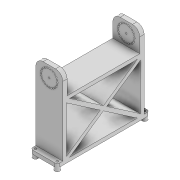
# Autodesk Inventor part: StereoVisionHolder
Saved by Autodesk Inventor 2022 (Build 260153000, 153)
## iProperties
Created: 2022-11-13
Part Number: StereoVisionHolder
Material: Generic
Document SubType Name: Modeling
Designer: MVeszpremi
Density: 1 g/cm^3
Appearance: Default
Author: MVeszpremi
Autodesk Inventor part; units mm, degrees
ref_plane "YZ Plane" through (0, 0, 0) normal (1, 0, 0) x (0, 1, 0)
ref_plane "XZ Plane" through (0, 0, 0) normal (0, 1, 0) x (-1, 0, 0)
ref_plane "XY Plane" through (0, 0, 0) normal (0, 0, 1) x (1, 0, 0)
sketch "Sketch1" plane through (0, 0, 0) normal (0, 1, 0) x (-1, 0, 0)
  line L0 (15, 60) -> (-15, 60)
  line L1 (-15, 60) -> (-15, -60)
  line L2 (-15, -60) -> (15, -60)
  line L3 (15, -60) -> (15, 60)
  line L4 (15, 60) -> (-15, -60) construction
  line L5 (-15, 60) -> (15, -60) construction
  circle A0 centre (15, 60) radius 3.5
  circle A1 centre (15, -60) radius 3.5
  circle A2 centre (-15, 60) radius 3.5
  circle A3 centre (-15, -60) radius 3.5
  circle A4 centre (15, 60) radius 1.5
  circle A5 centre (15, -60) radius 1.5
  circle A6 centre (-15, -60) radius 1.5
  circle A7 centre (-15, 60) radius 1.5
  line L6 (15, 63.5) -> (-15, 63.5)
  line L7 (-15, 63.5) -> (-15, -63.5)
  line L8 (-15, -63.5) -> (15, -63.5)
  line L9 (15, -63.5) -> (15, 63.5)
  line L10 (15, 63.5) -> (-15, -63.5) construction
  line L11 (-15, 63.5) -> (15, -63.5) construction
  line L12 (-18.5, -60) -> (18.5, -60)
  line L13 (18.5, -60) -> (18.5, 60)
  line L14 (18.5, 60) -> (-18.5, 60)
  line L15 (-18.5, 60) -> (-18.5, -60)
  line L16 (-18.5, -60) -> (18.5, 60) construction
  line L17 (18.5, -60) -> (-18.5, 60) construction
  point P0 (0, 0)
  point P1 (15, 56.5)
  point P2 (11.5, 60)
  point P3 (-11.5, 60)
  point P4 (-15, 56.5)
  point P5 (-15, -56.5)
  point P6 (-11.5, -60)
  point P7 (11.5, -60)
  point P8 (15, -56.5)
  point P9 (18.5, -60)
  dimension "d2" = 7
  dimension "d5" = 7
  dimension "d0" = 120
  dimension "d1" = 30
  dimension "d3" = 7
  dimension "d4" = 7
  dimension "d6" = 3
  dimension "d7" = 3
  dimension "d8" = 3
  dimension "d9" = 3
  constraints: 36 end point, 8 coincident, 6 centre point, 6 midpoint, 6 parallel, 3 horizontal, 3 perpendicular, 6 other
  measures "d0" distance of L2.end L0.start
  measures "d1" distance of L0.start L0.end
  measures "d3" diameter of A1
  measures "d4" diameter of A2
  measures "d6" diameter of A4
  measures "d7" diameter of A5
  measures "d8" diameter of A6
  measures "d9" diameter of A7
extrude "Extrusion1" add sketch "Sketch1" against normal blind 5 contours A2 L1 A7 L0 | L0 A7 L7 A2 | A0 L9 A4 L0 | L0 A4 L3 A0 | L7 A7 L14 A2 | A2 L14 A7 L1 | A0 L14 A4 L9 | L3 A4 L14 A0 | A3 L2 A6 L1 | L1 A6 L12 A3 | A1 L12 A5 L3 | L3 A5 L2 A1 | L12 A6 L7 A3 | A3 L7 A6 L2 | A1 L9 A5 L12 | L2 A5 L9 A1
extrude "Extrusion2" add sketch "Sketch1" along normal blind 5 contours A2 L1 A7 L0 | A2 L6 A0 L0 | L0 A7 L7 A2 | L0 A0 L3 A1 L2 A3 L1 A2 | A0 L9 A4 L0 | L0 A4 L3 A0 | L7 A7 L14 A2 | A2 L14 A7 L1 | L1 A3 L15 A2 | A0 L14 A4 L9 | A0 L13 A1 L3 | L3 A4 L14 A0 | A3 L2 A6 L1 | L1 A6 L12 A3 | A1 L12 A5 L3 | L3 A5 L2 A1 | L12 A6 L7 A3 | A3 L7 A6 L2 | L2 A1 L8 A3 | A1 L9 A5 L12 | L2 A5 L9 A1
sketch "Sketch8" plane through (0, 5, 0) normal (0, 1, 0) x (1, 0, 0)
  line L0 (-18.5, 60) -> (-18.5, -60) projected
  line L1 (18.5, -60) -> (18.5, 60) projected
  line L2 (-18.5, -56) -> (18.5, -56)
  line L3 (18.5, -56) -> (18.5, -51)
  line L4 (18.5, -51) -> (-18.5, -51)
  line L5 (-18.5, -51) -> (-18.5, -56)
  line L6 (-18.5, 51) -> (18.5, 51)
  line L7 (18.5, 51) -> (18.5, 56)
  line L8 (18.5, 56) -> (-18.5, 56)
  line L9 (-18.5, 56) -> (-18.5, 51)
  line L10 (-15, -63.5) -> (15, -63.5) projected
  line L11 (15, 63.5) -> (-15, 63.5) projected
  point P0 (0, 0)
  point P1 (18.5, -56)
  dimension "d37" = 5
  dimension "d38" = 7.5
  dimension "d39" = 5
  dimension "d40" = 7.5
  constraints: 16 end point, 4 parallel, 4 point on line, 2 horizontal, 2 perpendicular
  measures "d37" distance between parallel lines of L2 L4
  measures "d38" distance between parallel lines of L10 L2
  measures "d39" distance between parallel lines of L8 L6
  measures "d40" distance between parallel lines of L11 L8
extrude "Extrusion8" add sketch "Sketch8" along normal blind 75 contours L8 L1 L6 L0 | L4 L1 L2 L0
sketch "Sketch9" plane through (18.5, 0, 60) normal (1, 0, 0) x (0, 0, -1)
  line L0 (9, 5) -> (9, 80) projected
  line L1 (111, 5) -> (111, 80) projected
  line L2 (9, 80) -> (111, 80)
  line L3 (111, 80) -> (111, 75)
  line L4 (111, 75) -> (9, 75)
  line L5 (9, 75) -> (9, 80)
  line L6 (9, 75) -> (111, 5) construction
  line L7 (7.5854, 72.9387) -> (109.5854, 2.9387)
  line L8 (112.4146, 7.0613) -> (10.4146, 77.0613)
  arc A0 (10.4146, 77.0613) -> (7.5854, 72.9387) centre (9, 75) ccw
  arc A1 (109.5854, 2.9387) -> (112.4146, 7.0613) centre (111, 5) ccw
  line L9 (9, 5) -> (111, 5) projected
  line L10 (9, 5) -> (111, 75) construction
  line L11 (10.4146, 2.9387) -> (112.4146, 72.9387)
  line L12 (109.5854, 77.0613) -> (7.5854, 7.0613)
  arc A2 (7.5854, 7.0613) -> (10.4146, 2.9387) centre (9, 5) ccw
  arc A3 (112.4146, 72.9387) -> (109.5854, 77.0613) centre (111, 75) ccw
  point P0 (60, 0)
  point P1 (60, 40)
  point P2 (60, 40)
  point P3 (9, 77.5)
  point P4 (13.4182, 75)
  point P5 (106.5818, 75)
  point P6 (111, 77.5)
  point P7 (60, 43.0321)
  point P8 (9, 75)
  point P9 (9, 71.9679)
  point P10 (55.5818, 40)
  point P11 (9, 8.0321)
  point P12 (13.4182, 5)
  point P13 (60, 36.9679)
  point P14 (106.5818, 5)
  point P15 (111, 8.0321)
  point P16 (64.4182, 40)
  point P17 (111, 71.9679)
  dimension "d43" = 5
  dimension "d44" = 5
  dimension "d45" = 5
  constraints: 24 end point, 8 point on circle, 8 tangent, 4 centre point, 4 parallel, 2 midpoint, 1 horizontal, 1 perpendicular, 1 point on line
  measures "d43" distance between parallel lines of L4 L2
  measures "d44" distance between parallel lines of L11 L12
  measures "d45" distance between parallel lines of L7 L8
extrude "Extrusion9" add sketch "Sketch9" against normal up to surface (37 mm away) contours L0 L12 L7 L11 L9 | L0 L4 L8 L12 L7 | L12 L8 L11 L7 | L7 L11 L8 L1 L9 | L0 A0 L8 L4 | L12 L4 L1 L11 L8 | L0 L2 L1 A3 L12 L4 L8 A0 | L12 A3 L1 L4
sketch "Sketch10" plane through (0, 80, 0) normal (0, 1, 0) x (1, 0, 0)
  line L0 (18.5, -56) -> (-18.5, -56) projected
  line L1 (-18.5, 60) -> (-18.5, -60) projected
  line L2 (18.5, -56) -> (-18.5, -56)
  line L3 (-18.5, -56) -> (-18.5, -50)
  line L4 (-18.5, -50) -> (18.5, -50)
  line L5 (18.5, -50) -> (18.5, -56)
  line L6 (18.5, 56) -> (-18.5, 56) projected
  line L7 (18.5, 56) -> (-18.5, 56)
  line L8 (-18.5, 56) -> (-18.5, 50)
  line L9 (-18.5, 50) -> (18.5, 50)
  line L10 (18.5, 50) -> (18.5, 56)
  point P0 (0, 0)
  dimension "d48" = 6
  dimension "d49" = 6
  constraints: 16 end point, 4 parallel, 2 horizontal, 2 perpendicular, 2 point on line
  measures "d48" distance between parallel lines of L4 L0
  measures "d49" distance between parallel lines of L6 L9
extrude "Extrusion10" add sketch "Sketch10" along normal blind 30
sketch "Sketch11" plane through (18.5, 5, -56) normal (0, 0, -1) x (-1, 0, 0)
  line L0 (37, 105) -> (0, 105) projected
  line L1 (37, 75) -> (37, 105) projected
  line L2 (0, 105) -> (37, 105)
  line L3 (37, 105) -> (37, 75)
  line L4 (37, 75) -> (0, 75)
  line L5 (0, 75) -> (0, 105)
  line L6 (0, 75) -> (0, 105) projected
  line L7 (0, 75) -> (37, 105)
  circle A0 centre (18.5, 90) radius 11.25
  circle A1 centre (18.5, 101.25) radius 1
  circle A2 centre (15.5883, 100.8667) radius 1
  circle A3 centre (12.875, 99.7428) radius 1
  circle A4 centre (10.545, 97.955) radius 1
  circle A5 centre (8.7572, 95.625) radius 1
  circle A6 centre (7.6333, 92.9117) radius 1
  circle A7 centre (7.25, 90) radius 1
  circle A8 centre (7.6333, 87.0883) radius 1
  circle A9 centre (8.7572, 84.375) radius 1
  circle A10 centre (10.545, 82.045) radius 1
  circle A11 centre (12.875, 80.2572) radius 1
  circle A12 centre (15.5883, 79.1333) radius 1
  circle A13 centre (18.5, 78.75) radius 1
  circle A14 centre (21.4117, 79.1333) radius 1
  circle A15 centre (24.125, 80.2572) radius 1
  circle A16 centre (26.455, 82.045) radius 1
  circle A17 centre (28.2428, 84.375) radius 1
  circle A18 centre (29.3667, 87.0883) radius 1
  circle A19 centre (29.75, 90) radius 1
  circle A20 centre (29.3667, 92.9117) radius 1
  circle A21 centre (28.2428, 95.625) radius 1
  circle A22 centre (26.455, 97.955) radius 1
  circle A23 centre (24.125, 99.7428) radius 1
  circle A24 centre (21.4117, 100.8667) radius 1
  circle A25 centre (18.5, 90) radius 1
  line L8 (18.5, 90) -> (18.5, 105)
  line L9 (0, 105) -> (37, 105) projected
  point P0 (18.5, -5)
  dimension "d52" = 22.5
  dimension "d53" = 2
  dimension "d56" = 360
  dimension "d61" = 2
  constraints: 25 centre point, 12 end point, 2 midpoint, 2 parallel, 1 coincident, 1 horizontal, 1 perpendicular, 1 point on line, 1 vertical alignment, 51 other
  measures "d53" diameter of A1
  measures "d61" diameter of A25
extrude "Extrusion11" cut sketch "Sketch11" against normal blind 134.75 contours L8 A0 A1 | A1 A0 L8 | A25 L7 | L7 L8 A25 | A21 A0 | A0 A21 | A22 A0 | A0 A22 | A0 L8 A1 | A0 A1 L8 | L7 A25 L8 | A2 A0 | A0 A2 | A9 A0 | A0 A9 | A10 A0 | A0 A10 | A20 A0 | A0 A20 | A23 A0 | A0 A23 | A24 A0 | A0 A24 | A3 A0 | A0 A3 | A8 A0 | A0 A8 | A11 A0 | A0 A11 | A19 A0 | A0 A19 | A4 A0 | A0 A4 | A7 A0 | A0 A7 | A12 A0 | A0 A12 | A18 A0 | A0 A18 | A5 A0 | A0 A5 | A6 A0 | A0 A6 | A13 A0 | A0 A13 | A17 A0 | A0 A17 | A14 A0 | A0 A14 | A16 A0 | A0 A16 | A15 A0 | A0 A15
fillet "Fillet1" radius 10 4 edges at (-18.5, 110, 53) (18.5, 110, 53) (-18.5, 110, -53) (18.5, 110, -53)
sketch "Sketch12" plane through (-18.5, 5, 56) normal (0, 0, 1) x (1, 0, 0)
  point P0 (18.5, -5)
body "Solid1"
